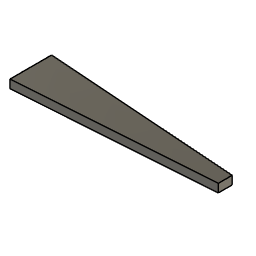
Main Wing (Autodesk Fusion 360 design; units mm, degrees)
Autodesk Fusion 360 part; units mm, degrees
sketch "Sketch1" plane through (0, 0, 0) normal (0, 0, 1) x (1, 0, 0)
  line L0 (0, 0) -> (0, 1500)
  line L1 (0, 1500) -> (7000, 1000)
  line L2 (0, 0) -> (7000, 500)
  line L3 (7000, 500) -> (7000, 1000)
  constraint coincident L0.start L2.start
  constraint vertical L0
  constraint parallel L0 L3
extrude "Extrude1" add sketch "Sketch1" against normal blind 300
